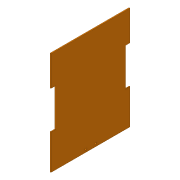
# Autodesk Inventor part: BackFlap
Saved by Autodesk Inventor 2016 (Build 200138000, 138)
## iProperties
Created: 2016-04-01
Part Number: BackFlap
Material: Generic
Document SubType Name: Modeling
Designer: aoben3
Density: 1 g/cm^3
Appearance: Orange
Author: aoben3
Autodesk Inventor part; units mm, degrees
ref_plane "YZ Plane" through (0, 0, 0) normal (1, 0, 0) x (0, 1, 0)
ref_plane "XZ Plane" through (0, 0, 0) normal (0, 1, 0) x (-1, 0, 0)
sketch "Sketch1" plane through (0, 0, 0) normal (1, 0, 0) x (0, 1, 0)
  line L0 (147.32, 113.03) -> (-147.32, 113.03)
  line L1 (-147.32, 113.03) -> (-147.32, -113.03)
  line L2 (-147.32, -113.03) -> (147.32, -113.03)
  line L3 (147.32, -113.03) -> (147.32, 113.03)
  line L4 (147.32, 113.03) -> (-147.32, -113.03) construction
  line L5 (-147.32, 113.03) -> (147.32, -113.03) construction
  point P0 (0, 0)
  dimension "d0" = 294.64
  dimension "d1" = 226.06
  constraints: 12 end point, 2 midpoint, 2 parallel, 1 horizontal, 1 perpendicular
  measures "d0" distance of L1.end L2.end
  measures "d1" distance of L2.end L0.start
extrude "Extrusion1" add sketch "Sketch1" along normal blind 2.8575
sketch "Sketch2" plane through (2.8575, 0, 0) normal (1, 0, 0) x (0, 0, -1)
  line L0 (113.03, 60.96) -> (100.33, 60.96)
  line L1 (100.33, 60.96) -> (100.33, -46.99)
  line L2 (100.33, -46.99) -> (113.03, -46.99)
  line L3 (113.03, -147.32) -> (113.03, 147.32) projected
  line L4 (113.03, 147.32) -> (-113.03, 147.32) projected
  line L5 (113.03, 60.96) -> (113.03, -46.99)
  point P0 (0, 0)
  dimension "d4" = 107.95
  dimension "d5" = 0
  dimension "d6" = 0
  dimension "d7" = 12.7
  dimension "d8" = 86.36
  constraints: 8 end point, 2 perpendicular, 1 horizontal
  measures "d4" distance of L0.end L1.end
  measures "d5" horizontal distance of L2.end L0.start
  measures "d6" distance from line of L3 L0.start
  measures "d7" distance of L0.start L0.end
  measures "d8" distance between parallel lines of L4 L0
extrude "Extrusion2" cut sketch "Sketch2" against normal blind 2.8575
mirror "Mirror1" about plane through (0, 0, 0) normal (0, 0, 1) of "Extrusion2"
ref_plane "Work Plane1" through (9.2075, 0, 0) normal (1, 0, 0) x (0, 0, -1)
fillet "Fillet2" radius 0.762 12 edges at (0, 104.14, -113.03) (0, 6.985, -100.33) (0, 60.96, -106.68) (0, -97.155, -113.03) (0, -46.99, -106.68) (0, -147.32, 0) (0, -97.155, 113.03) (0, -46.99, 106.68) (0, 6.985, 100.33) (0, 60.96, 106.68) (0, 104.14, 113.03) (2.8575, 147.32, 0)
fillet "Fillet4" radius 0.254 18 edges at (2.8575, -147.32, 0) (2.8575, -97.155, -113.03) (2.8575, 6.985, -100.33) (2.8575, -46.99, -106.68) (2.6343, 147.0968, -113.03) (1.4287, 147.32, -113.03) (0.2232, 147.32, -112.8068) (0, 147.32, 0) (0.2232, 147.32, 112.8068) (1.4287, 147.32, 113.03) (2.6343, 147.0968, 113.03) (2.8575, 103.759, 113.03) (2.8575, 103.759, -113.03) (2.8575, 60.96, -106.68) (2.8575, 60.96, 106.68) (2.8575, 6.985, 100.33) (2.8575, -97.155, 113.03) (2.8575, -46.99, 106.68)
sketch "Sketch7" plane through (0, 0, 0) normal (-1, 0, 0) x (0, 0, 1)
  circle A0 centre (-13.97, -138.938) radius 2.54
  line L0 (0, 0) -> (0, -146.558) construction
  line L1 (112.268, -146.558) -> (-112.268, -146.558) projected
  circle A1 centre (13.97, -138.938) radius 2.54
  dimension "d22" = 5.08
  dimension "d23" = 13.97
  dimension "d24" = 7.62
  constraints: 2 centre point, 2 end point, 1 coincident, 1 midpoint, 1 symmetric about line, 1 vertical, 1 other
  measures "d22" diameter of A0
  measures "d23" distance from line of A0.centre L0
  measures "d24" distance from line of A0.centre L1
extrude "Extrusion4" cut sketch "Sketch7" against normal up to next
body "Solid1"
